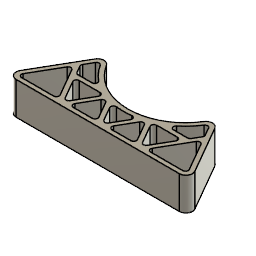
VOLT_Cradle v3 (Autodesk Fusion 360 design; units mm, degrees)
Autodesk Fusion 360 part; units mm, degrees
sketch "Sketch1" plane through (0, 0, 0) normal (0, 1, 0) x (1, 0, 0)
  circle A0 centre (0, 0) radius 68.2625 construction
  line L0 (0, 0) -> (0, -72.136) construction
  circle A1 centre (0, -72.136) radius 22.098 construction
  circle A2 centre (0, 0) radius 65.7225 construction
  circle A3 centre (0, 0) radius 66.3575
  line L1 (0, -72.136) -> (0, -101.6) construction
  line L2 (-107.95, -101.6) -> (107.95, -101.6)
  line L3 (-107.95, -101.6) -> (-62.3707, -22.6543)
  line L4 (107.95, -101.6) -> (62.3707, -22.6543)
  circle A4 centre (0, 0) radius 71.4375
  line L5 (-62.9376, -33.7962) -> (-99.1512, -96.52)
  line L6 (-99.1512, -96.52) -> (99.1512, -96.52)
  line L7 (99.1512, -96.52) -> (59.9049, -28.5434)
  line L8 (0, -96.52) -> (15.4586, -69.7449)
  line L9 (5.8659, -96.52) -> (22.4337, -67.8236)
  line L10 (22.4337, -67.8236) -> (39.0016, -96.52)
  line L11 (44.8675, -96.52) -> (27.2642, -66.0302)
  line L12 (44.8675, -96.52) -> (72.0093, -49.5089)
  line L13 (50.7334, -96.52) -> (74.9423, -54.5889)
  line L14 (27.2642, -66.0302) -> (62.4708, -66.0302)
  line L15 (37.2612, -60.9502) -> (65.4037, -60.9502)
  line L16 (0, -96.52) -> (-15.4586, -69.7449)
  line L17 (-22.4337, -67.8236) -> (-39.0016, -96.52)
  line L18 (-5.8659, -96.52) -> (-22.4337, -67.8236)
  line L19 (-44.8675, -96.52) -> (-27.2642, -66.0302)
  line L20 (-27.2642, -66.0302) -> (-62.4708, -66.0302)
  line L21 (-44.8675, -96.52) -> (-72.0093, -49.5089)
  line L22 (-50.7334, -96.52) -> (-74.9423, -54.5889)
  line L23 (-37.2612, -60.9502) -> (-65.4037, -60.9502)
  dimension "d1" = 136.525
  dimension "d2" = 72.136
  dimension "d3" = 44.196
  dimension "d7" = 131.445
  dimension "d8" = 0.635
  dimension "d9" = 101.6
  dimension "d10" = 60
  dimension "d11" = 215.9
  dimension "d14" = 5.08
  dimension "d15" = 5.08
  dimension "d16" = 5.08
  dimension "d17" = 5.08
  dimension "d30" = 30
  dimension "d31" = 5.08
  dimension "d32" = 60
  dimension "d34" = 60
  dimension "d35" = 5.08
  dimension "d36" = 5.08
  dimension "d37" = 5.08
  constraint coincident A0.centre L0.start
  constraint vertical L0
  constraint coincident L0.end A1.centre
  constraint concentric A2 A3
  constraint parallel L0 L1
  constraint horizontal L2
  constraint midpoint L1.end L2
  constraint coincident A3 L3.end
  constraint symmetric L0 L2.start L2.end
  constraint symmetric L0 L3.end L4.end
  constraint coincident A4 L5.start
  constraint parallel L3 L5
  constraint perpendicular L1 L6
  constraint coincident A3 L7.end
  constraint parallel L4 L7
  constraint midpoint L6 L8.start
  constraint coincident A4 L8.end
  constraint coincident L6 L9.start
  constraint coincident A4 L9.end
  constraint parallel L8 L9
  constraint coincident L6 L10.end
  constraint coincident L6 L11.start
  constraint coincident A4 L11.end
  constraint parallel L10 L11
  constraint coincident L7 L12.end
  constraint coincident L6 L13.start
  constraint coincident L7 L13.end
  constraint parallel L12 L13
  constraint coincident L12 L14.end
  constraint horizontal L14
  constraint coincident A4 L15.start
  constraint coincident L12 L15.end
  constraint parallel L14 L15
  constraint symmetric L1 L8.start L16.start
  constraint symmetric L1 L8.end L16.end
  constraint symmetric L1 L9.start L18.start
  constraint symmetric L1 L9.end L17.start
  constraint symmetric L1 L10.end L17.end
  constraint symmetric L1 L11.start L19.start
  constraint symmetric L1 L11.end L19.end
  constraint symmetric L1 L12.end L21.end
  constraint symmetric L1 L13.start L22.start
  constraint symmetric L1 L13.end L22.end
  constraint symmetric L1 L14.end L20.end
  constraint symmetric L1 L15.start L23.start
  constraint symmetric L1 L15.end L23.end
  measures "d1" diameter of A0
  measures "d2" distance of A0.centre L0.end
  measures "d3" diameter of A1
  measures "d7" diameter of A2
  measures "d8" distance of A2 A3
  measures "d9" distance of A0.centre L2
  measures "d10" angle of L2 L3
  measures "d11" distance of L2.start L2.end
  measures "d14" distance of A3 A4
  measures "d15" distance of L3 L5
  measures "d16" distance of L2 L6
  measures "d17" distance of L4 L7
  measures "d30" angle of L1 L8
  measures "d31" distance of L8 L9
  measures "d32" angle of L9 L10
  measures "d34" angle of L11 L12
  measures "d35" distance of L10 L11
  measures "d36" distance of L12 L13
  measures "d37" distance of L14 L15
extrude "Extrude1" add sketch "Sketch1" along normal blind 38.1 contours A3 L3 A4 L7 | A3 L4 A4 L7 | L2 L3 L4 A4 L5 L6 L7 | A4 L12 L14 L15 | L6 L7 L12 L13 | A4 L20 L21 L23 | L5 L6 L21 L22 | A4 L6 L10 L11 | A4 L6 L17 L19 | A4 L6 L8 L9 | A4 L6 L16 L18
fillet "Fillet2" radius 3.175 29 edges at (-62.9376, 19.05, 33.7962) (-99.1512, 19.05, 96.52) (99.1512, 19.05, 96.52) (62.9376, 19.05, 33.7962) (-72.0093, 19.05, 49.5089) (-65.4037, 19.05, 60.9502) (-37.2612, 19.05, 60.9502) (-74.9423, 19.05, 54.5889) (-50.7334, 19.05, 96.52) (-62.4708, 19.05, 66.0302) (-44.8675, 19.05, 96.52) (-27.2642, 19.05, 66.0302) (-39.0016, 19.05, 96.52) (-22.4337, 19.05, 67.8236) (-5.8659, 19.05, 96.52) (-15.4586, 19.05, 69.7449) (15.4586, 19.05, 69.7449) (0, 19.05, 96.52) (5.8659, 19.05, 96.52) (22.4337, 19.05, 67.8236) (39.0016, 19.05, 96.52) (27.2642, 19.05, 66.0302) (44.8675, 19.05, 96.52) (62.4708, 19.05, 66.0302) (37.2612, 19.05, 60.9502) (72.0093, 19.05, 49.5089) (65.4037, 19.05, 60.9502) (74.9423, 19.05, 54.5889) (50.7334, 19.05, 96.52)
fillet "Fillet1" radius 7.62 4 edges at (-62.3707, 19.05, 22.6543) (62.3707, 19.05, 22.6543) (107.95, 19.05, 101.6) (-107.95, 19.05, 101.6)
equation "d15 = d14"
equation "d16 = d14"
equation "d17 = d14"
equation "d31 = d14"
equation "d35 = d14"
equation "d36 = d35"
equation "d37 = d17"
